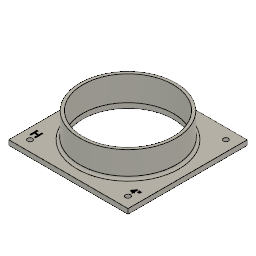
To 4_ Flex Hose (Autodesk Fusion 360 design; units mm, degrees)
Autodesk Fusion 360 part; units mm, degrees
sketch "Sketch1" plane through (0, 0, 0) normal (0, 1, 0) x (1, 0, 0)
  circle A0 centre (0, 0) radius 44.8125
  circle A1 centre (0, 0) radius 47.8125
  line L0 (59, 59) -> (-59, 59)
  line L1 (-59, 59) -> (-59, -59)
  line L2 (-59, -59) -> (59, -59)
  line L3 (59, -59) -> (59, 59)
  line L4 (59, 59) -> (-59, -59) construction
  line L5 (-59, 59) -> (59, -59) construction
  circle A2 centre (-48.3934, 48.3934) radius 2.5
  circle A3 centre (-48.3934, -48.3934) radius 2.5
  circle A4 centre (48.3934, -48.3934) radius 2.5
  circle A5 centre (48.3934, 48.3934) radius 2.5
  dimension "d7" = 89.625
  dimension "d8" = 95.625
  dimension "d9" = 118
  dimension "d10" = 118
  dimension "d11" = 5
  dimension "d12" = 15
  dimension "d15" = 0
  dimension "d16" = 0
  dimension "d18" = 360
  measures "d7" diameter of A0
  measures "d8" diameter of A1
  measures "d11" diameter of A2
ref_plane "WorkPlane1" through (0, 30, 0) normal (0, 1, 0) x (1, 0, 0)
sketch "Sketch2" plane through (0, 30, 0) normal (0, 1, 0) x (1, 0, 0)
  circle A0 centre (0, 0) radius 44.4375
  circle A1 centre (0, 0) radius 47.4375
  dimension "d20" = 88.875
  dimension "d21" = 94.875
  measures "d20" diameter of A0
  measures "d21" diameter of A1
extrude "Extrude1" add sketch "Sketch1" along normal blind 5 contours A1 | L0 L1 L2 L3
ref_plane "WorkPlane2" through (0, 5, 0) normal (0, 1, 0) x (1, 0, 0)
sketch "Sketch3" plane through (0, 5, 0) normal (0, 1, 0) x (1, 0, 0)
  line L0 (59, -59) -> (59, 59)
  circle A0 centre (0, 0) radius 47.8125
  circle A1 centre (0, 0) radius 44.8125
  line L1 (-59, 59) -> (59, -59) construction
  dimension "d25" = 89.625
  dimension "d26" = 95.625
  measures "d25" diameter of A1
  measures "d26" diameter of A0
loft "Loft1" add profiles "Sketch2", "Sketch3" section 1 section 2
loft "Loft2" cut profiles "Sketch2", "Sketch3" section 1 contours A0 section 2 contours A1
fillet "Fillet2" radius 2.5 1 edges at (-44.5769, 5, -17.2897)
sketch "Sketch4" plane through (0, 0, 0) normal (0, 0, 1) x (1, 0, 0)
  line L0 (0, 17) -> (25.7422, 17) construction
  line L1 (25.7422, 17) -> (25.7422, 27) construction
  line L2 (25.7422, 27) -> (0, 27) construction
  line L3 (0, 27) -> (0, 17) construction
sketch "Sketch5" plane through (0, 5, 0) normal (0, 1, 0) x (-1, 0, 0)
  line L0 (-59, 59) -> (-59, -59)
  line L1 (-59, -59) -> (59, -59)
  line L2 (59, -59) -> (59, 59)
  line L3 (59, 59) -> (-59, 59)
  circle A0 centre (48.3934, -48.3934) radius 2.5
  circle A1 centre (-48.3934, -48.3934) radius 2.5
  circle A2 centre (-48.3934, 48.3934) radius 2.5
  circle A3 centre (48.3934, 48.3934) radius 2.5
  circle A4 centre (0, 0) radius 50.2753
  line L4 (53, 44) -> (47.3848, 44) construction
  line L5 (47.3848, 44) -> (47.3848, 34) construction
  line L6 (47.3848, 34) -> (53, 34) construction
  line L7 (53, 34) -> (53, 44) construction
  text T0 "H" font "Arial" height 10 align ink ink in box 0 x 0 at (53, 44) x (-1, 0) y (0, -1) spacing 1 height is em
extrude "Extrude2" cut sketch "Sketch5" against normal blind 0.5 text T0
sketch "Sketch6" plane through (0, 5, 0) normal (0, 1, 0) x (-1, 0, 0)
  line L0 (48.322, 43.99) -> (48.322, 40.616)
  line L1 (48.322, 40.616) -> (52.0427, 40.616)
  line L2 (52.99, 43.99) -> (52.99, 36.8318)
  line L3 (52.99, 36.8318) -> (52.0427, 36.8318)
  line L4 (52.0427, 36.8318) -> (52.0427, 39.7713)
  line L5 (52.0427, 39.7713) -> (48.322, 39.7713)
  line L6 (48.322, 39.7713) -> (48.322, 36.8318)
  line L7 (48.322, 36.8318) -> (47.3748, 36.8318)
  line L8 (47.3748, 36.8318) -> (47.3748, 43.99)
  line L9 (47.3748, 43.99) -> (48.322, 43.99)
  line L10 (-59, 59) -> (-59, -59)
  line L11 (-59, -59) -> (59, -59)
  line L12 (59, -59) -> (59, 59)
  line L13 (59, 59) -> (-59, 59)
  circle A0 centre (48.3934, -48.3934) radius 2.5
  circle A1 centre (-48.3934, -48.3934) radius 2.5
  circle A2 centre (-48.3934, 48.3934) radius 2.5
  circle A3 centre (48.3934, 48.3934) radius 2.5
  circle A4 centre (0, 0) radius 50.2753
  line L14 (-44.63, 43.87) -> (-51.4425, 43.87) construction
  line L15 (-51.4425, 43.87) -> (-51.4425, 35.87) construction
  line L16 (-51.4425, 35.87) -> (-44.63, 35.87) construction
  line L17 (-44.63, 35.87) -> (-44.63, 43.87) construction
  line L18 (52.0427, 40.616) -> (52.0427, 43.99)
  line L19 (52.0427, 43.99) -> (52.99, 43.99)
  text T0 "4\"" font "Arial" height 8 align ink ink in box 0 x 0 at (-44.63, 43.87) x (-1, 0) y (0, -1) spacing 1 height is em
extrude "Extrude3" cut sketch "Sketch6" against normal blind 0.5 text T0
equation "ID = OD - ( WallThickness * 2 )"
equation "OD = 3.75 in"
equation "WallThickness = 3 mm"
equation "Length = 30 mm"
equation "ScrewHoleDiam = 5 mm"
equation "TaperOffset = 0.75 mm"
equation "d7 = ID + ( TaperOffset / 2 )"
equation "d8 = OD + ( TaperOffset / 2 )"
equation "d11 = ScrewHoleDiam"
equation "d19 = Length"
equation "d20 = ID - ( TaperOffset / 2 )"
equation "d21 = OD - ( TaperOffset / 2 )"
equation "d25 = ID + ( TaperOffset / 2 )"
equation "d26 = OD + ( TaperOffset / 2 )"
